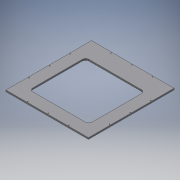
# Autodesk Inventor part: Låg mk2
Saved by Autodesk Inventor 2016 (Build 200138000, 138)
## iProperties
Created: 2015-10-19
Part Number: Låg mk2
Material: Generic
Document SubType Name: Modeling
Designer: iLyngklip
Density: 1 g/cm^3
Appearance: Default
Author: iLyngklip
Autodesk Inventor part; units mm, degrees
ref_plane "YZ Plane" through (0, 0, 0) normal (1, 0, 0) x (0, 1, 0)
ref_plane "XZ Plane" through (0, 0, 0) normal (0, 1, 0) x (-1, 0, 0)
ref_plane "XY Plane" through (0, 0, 0) normal (0, 0, 1) x (1, 0, 0)
sketch "Sketch1" plane through (0, 0, 0) normal (0, 0, 1) x (1, 0, 0)
  line L0 (-160, 166) -> (160, 166)
  line L1 (160, 166) -> (160, -166)
  line L2 (160, -166) -> (-160, -166)
  line L3 (-160, -166) -> (-160, 166)
  point P0 (0, 0)
  dimension "d0" = 320
  dimension "d1" = 332
  dimension "d2" = 160
  dimension "d3" = 166
  constraints: 8 end point, 2 parallel, 1 horizontal, 1 perpendicular
  measures "d0" distance of L1.end L2.end
  measures "d1" distance of L0.end L1.end
  measures "d2" distance from line of point (0, 0) L1
  measures "d3" distance from line of point (0, 0) L2
extrude "Tykkelse" add sketch "Sketch1" along normal mid plane 6
sketch "Sketch2" plane through (0, 0, 3) normal (0, 0, 1) x (1, 0, 0)
  line L0 (-102, 98) -> (102, 98)
  line L1 (115, 85) -> (115, -107)
  line L2 (102, -120) -> (-102, -120)
  line L3 (-115, -107) -> (-115, 85)
  line L4 (160, -166) -> (160, 166) projected
  line L5 (-160, 166) -> (-160, -166) projected
  line L6 (-160, -166) -> (160, -166) projected
  line L7 (160, 166) -> (-160, 166) projected
  arc A0 (-102, 98) -> (-115, 85) centre (-102, 85) ccw
  arc A1 (115, 85) -> (102, 98) centre (102, 85) ccw
  arc A2 (102, -120) -> (115, -107) centre (102, -107) ccw
  arc A3 (-115, -107) -> (-102, -120) centre (-102, -107) ccw
  point P0 (0, 0)
  dimension "d6" = 45
  dimension "d7" = 45
  dimension "d8" = 46
  dimension "d9" = 68
  dimension "d10" = 13
  dimension "d20" = 218
  dimension "d21" = 230
  constraints: 8 end point, 8 point on circle, 8 tangent, 4 centre point, 3 equal radius, 2 parallel, 1 horizontal, 1 perpendicular
  measures "d6" distance between parallel lines of L4 L1
  measures "d7" distance between parallel lines of L5 L3
  measures "d8" distance between parallel lines of L6 L2
  measures "d9" distance between parallel lines of L7 L0
  measures "d10" radius of A0
  measures "d20" distance between parallel lines of L0 L2
  measures "d21" distance between parallel lines of L3 L1
extrude "Vindue" cut sketch "Sketch2" against normal up to surface (6 mm away) contours L0 A1 L1 A2 L2 A3 L3 A0
sketch "Sketch3" plane through (0, 0, -3) normal (0, 0, -1) x (-1, 0, 0)
  circle A0 centre (65, 138) radius 6
  circle A1 centre (-65, 138) radius 6
  line L0 (-65, 138) -> (65, 138) construction
  line L1 (160, 166) -> (-160, 166) projected
  point P0 (0, 0)
  dimension "d13" = 12
  dimension "d14" = 12
  dimension "d15" = 130
  dimension "d16" = 65
  dimension "d17" = 28
  constraints: 2 centre point, 2 end point, 1 horizontal
  measures "d13" diameter of A1
  measures "d14" diameter of A0
  measures "d15" distance of L0.start L0.end
  measures "d16" horizontal distance of point (0, 0) L0.start
  measures "d17" distance between parallel lines of L1 L0
extrude "Ø12 mm huller" cut sketch "Sketch3" against normal blind 3.5
sketch "Sketch4" plane through (0, 0, 3) normal (0, 0, 1) x (1, 0, 0)
  line L0 (156, 162) -> (-156, 162) construction
  line L1 (-156, 162) -> (-156, -162) construction
  line L2 (-156, -162) -> (156, -162) construction
  line L3 (156, -162) -> (156, 162) construction
  circle A0 centre (-156, -80) radius 1.5
  circle A1 centre (-156, 0) radius 1.5
  circle A2 centre (-156, 80) radius 1.5
  circle A3 centre (-80, 162) radius 1.5
  circle A4 centre (0, 162) radius 1.5
  circle A5 centre (80, 162) radius 1.5
  circle A6 centre (156, 80) radius 1.5
  circle A7 centre (156, 0) radius 1.5
  circle A8 centre (156, -80) radius 1.5
  circle A9 centre (-80, -162) radius 1.5
  circle A10 centre (0, -162) radius 1.5
  circle A11 centre (80, -162) radius 1.5
  line L4 (-160, 166) -> (-160, -166) construction
  line L5 (-160, -166) -> (160, -166) construction
  line L6 (160, 166) -> (-160, 166) construction
  line L7 (160, -166) -> (160, 166) construction
  point P0 (0, 0)
  dimension "d22" = 3
  dimension "d23" = 3
  dimension "d24" = 3
  dimension "d25" = 3
  dimension "d26" = 3
  dimension "d27" = 3
  dimension "d28" = 3
  dimension "d29" = 3
  dimension "d30" = 3
  dimension "d31" = 3
  dimension "d32" = 3
  dimension "d33" = 3
  dimension "d34" = 4
  dimension "d35" = 4
  dimension "d36" = 4
  dimension "d37" = 4
  dimension "d38" = 240
  dimension "d39" = 160
  dimension "d40" = 80
  dimension "d41" = 80
  dimension "d42" = 160
  dimension "d43" = 240
  dimension "d44" = 86
  dimension "d45" = 166
  dimension "d46" = 246
  dimension "d47" = 246
  dimension "d48" = 166
  dimension "d49" = 86
  constraints: 12 centre point, 8 end point, 8 point on line, 4 midpoint, 2 parallel, 1 horizontal, 1 perpendicular
  measures "d22" diameter of A2
  measures "d23" diameter of A0
  measures "d24" diameter of A1
  measures "d25" diameter of A3
  measures "d26" diameter of A4
  measures "d27" diameter of A5
  measures "d28" diameter of A6
  measures "d29" diameter of A7
  measures "d30" diameter of A8
  measures "d31" diameter of A9
  measures "d32" diameter of A10
  measures "d33" diameter of A11
  measures "d34" distance between parallel lines of L4 L1
  measures "d35" distance between parallel lines of L5 L2
  measures "d36" distance between parallel lines of L6 L0
  measures "d37" distance between parallel lines of L7 L3
  measures "d38" distance from line of A9.centre L7
  measures "d39" distance from line of A10.centre L7
  measures "d40" distance from line of L7 A11.centre
  measures "d41" distance from line of L7 A5.centre
  measures "d42" distance from line of L7 A4.centre
  measures "d43" distance from line of L7 A3.centre
  measures "d44" distance from line of A2.centre L6
  measures "d45" distance from line of A1.centre L6
  measures "d46" distance from line of L6 A0.centre
  measures "d47" distance from line of L6 A8.centre
  measures "d48" distance from line of L6 A7.centre
  measures "d49" distance from line of L6 A6.centre
extrude "Monteringshuller" cut sketch "Sketch4" against normal up to surface (6 mm away)
equation "\"d2\" = 0.5 * d0"
equation "\"d3\" = 0.5 * d1"
equation "\"d7\" = d6"
equation "\"d14\" = d13"
equation "\"d16\" = 0.5 * d15"
equation "\"d22\" = d23"
equation "\"d24\" = d23"
equation "\"d25\" = d23"
equation "\"d26\" = d23"
equation "\"d27\" = d23"
equation "\"d28\" = d23"
equation "\"d29\" = d23"
equation "\"d30\" = d23"
equation "\"d31\" = d23"
equation "\"d32\" = d23"
equation "\"d33\" = d23"
body "Solid1"
